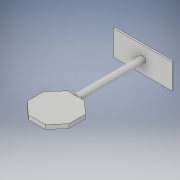
# Autodesk Inventor part: Stoppschild
Saved by Autodesk Inventor 2019.5 (Build 235369000, 369)
## iProperties
Created: 2021-09-30
Part Number: Stoppschild
Material: Generisch
Document SubType Name: Modeling
Designer: mritt
Density: 1 g/cm^3
Appearance: Vorgabe
Author: mritt
Autodesk Inventor part; units mm, degrees
ref_plane "YZ Plane" through (0, 0, 0) normal (1, 0, 0) x (0, 1, 0)
ref_plane "XZ Plane" through (0, 0, 0) normal (0, 1, 0) x (-1, 0, 0)
ref_plane "XY Plane" through (0, 0, 0) normal (0, 0, 1) x (1, 0, 0)
sketch "Skizze1" plane through (0, 0, 0) normal (0, 1, 0) x (-1, 0, 0)
  line L0 (35.5112, -88.3128) -> (35.5112, -108.3128)
  line L1 (35.5112, -108.3128) -> (22.0645, -123.1178)
  line L2 (22.0645, -123.1178) -> (2.0645, -123.1178)
  line L3 (2.0645, -123.1178) -> (-12.7404, -109.6711)
  line L4 (-12.7404, -109.6711) -> (-12.7404, -89.6711)
  line L5 (-12.7404, -89.6711) -> (0.7063, -74.8661)
  line L6 (0.7063, -74.8661) -> (20.7063, -74.8661)
  line L7 (20.7063, -74.8661) -> (35.5112, -88.3128)
  point P0 (0, 0)
  dimension "d0" = 20
  dimension "d1" = 20
  dimension "d2" = 20
  dimension "d3" = 20
  dimension "d4" = 20
  dimension "d5" = 20
  dimension "d6" = 20
  dimension "d7" = 20
  constraints: 16 end point, 2 parallel, 2 perpendicular, 1 vertical
  measures "d0" distance of L0.start L0.end
  measures "d1" distance of L3.end L4.end
  measures "d2" distance of L1.end L2.end
  measures "d3" distance of L5.end L6.end
  measures "d4" distance of L0.end L1.end
  measures "d5" distance of L6.end L0.start
  measures "d6" distance of L2.end L3.end
  measures "d7" distance of L4.end L5.end
extrude "Extrusion1" add sketch "Skizze1" along normal blind 5
sketch "Skizze2" plane through (-2.0645, 0, -123.1178) normal (0, 0, -1) x (-1, 0, 0)
  circle A0 centre (10, 2.5) radius 3.75
  line L0 (0, 5) -> (20, 5) projected
  point P0 (-2.0645, 0)
  dimension "d11" = 7.5
  dimension "d12" = 2.5
  constraints: 1 centre point
  measures "d11" diameter of A0
  measures "d12" distance from line of A0.centre L0
extrude "Extrusion2" add sketch "Skizze2" along normal blind 81.748
sketch "Skizze3" plane through (-12.0645, 2.5, -204.8658) normal (0, 0, -1) x (-1, 0, 0)
  line L0 (-35, -15) -> (35, -15)
  line L1 (35, -15) -> (35, 15)
  line L2 (35, 15) -> (-35, 15)
  line L3 (-35, 15) -> (-35, -15)
  arc A0 (-2.7951, 2.5) -> (-2.7951, -2.5) centre (0, 0) ccw projected
  line L4 (-35, -15) -> (35, 15) construction
  line L5 (35, -15) -> (-35, 15) construction
  point P0 (-12.0645, -2.5)
  dimension "d15" = 70
  dimension "d16" = 30
  constraints: 12 end point, 2 midpoint, 2 parallel, 1 horizontal, 1 perpendicular
  measures "d15" distance of L1.end L2.end
  measures "d16" distance of L0.end L1.end
extrude "Extrusion3" add sketch "Skizze3" against normal blind 2
